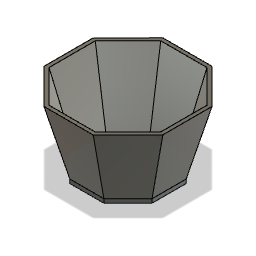
MacetaFinal (Autodesk Fusion 360 design; units mm, degrees)
Autodesk Fusion 360 part; units mm, degrees
sketch "Boceto2" plane through (0, 0, 0) normal (0, 1, 0) x (1, 0, 0)
  line L0 (0, 0) -> (35, 0)
  line L1 (35, 0) -> (59.7299, -24.7676)
  line L2 (59.7299, -24.7676) -> (59.7299, -59.7676)
  line L3 (59.7299, -59.7676) -> (34.9925, -84.5277)
  line L4 (34.9925, -84.5277) -> (-0.0075, -84.5277)
  line L5 (-0.0075, -84.5277) -> (-24.7562, -59.779)
  line L6 (-24.7562, -59.779) -> (-24.7562, -24.779)
  line L7 (0, 0) -> (-24.7562, -24.779)
  dimension "d12" = 35
  dimension "d16" = 35
  constraint coincident L0.start L7.start
  constraint horizontal L0
  constraint vertical L2
  constraint perpendicular L2 L4
  constraint vertical L6
  measures "d12" distance of L0.start L0.end
  measures "d16" distance of L3.end L4.end
extrude "Extruir1" add sketch "Boceto2" along normal blind 70 draft 15
sketch "Boceto3" plane through (0, 0, 0) normal (0, 0, 1) x (1, 0, 0)
  line L0 (33.4625, 0, 80.8319) -> (56.0342, 0, 58.2371)
  line L1 (56.0346, 0, 26.2989) -> (56.0342, 0, 58.2371)
  line L2 (56.0346, 0, 26.2989) -> (33.4695, 0, 3.6956)
  line L3 (33.4695, 0, 3.6956) -> (1.53, 0, 3.6958)
  line L4 (-21.0606, 0, 26.3095) -> (1.53, 0, 3.6958)
  line L5 (-21.0606, 0, 26.3095) -> (-21.061, 0, 58.2476)
  line L6 (-21.061, 0, 58.2476) -> (1.5231, 0, 80.8321)
  line L7 (1.5231, 0, 80.8321) -> (33.4625, 0, 80.8319)
  point P0 (34.9925, 0)
  point P1 (59.7299, 0)
  point P2 (-24.7562, 0)
  point P3 (-0.0075, 0)
  point P4 (35, 0)
  point P5 (59.7299, 0)
  point P6 (-24.7562, 0)
  dimension "d26" = 4
  dimension "d27" = 4
  dimension "d30" = 4
  dimension "d31" = 4
extrude "Extruir2" cut sketch "Boceto3" along normal blind 80 draft 15 contours L0 L1 L2 L3 L4 L5 L6 L7 in plane through (0, 0, 0) normal (0, 1, 0)
sketch "Boceto4" plane through (0, 0, 0) normal (0, -1, 0) x (1, 0, 0)
  line L0 (1.53, 3.6958) -> (-21.0606, 26.3095)
  line L1 (-21.0606, 26.3095) -> (-21.061, 58.2476)
  line L2 (-21.061, 58.2476) -> (1.5231, 80.8321)
  line L3 (1.5231, 80.8321) -> (33.4625, 80.8319)
  line L4 (33.4625, 80.8319) -> (56.0342, 58.2371)
  line L5 (56.0342, 58.2371) -> (56.0346, 26.2989)
  line L6 (56.0346, 26.2989) -> (33.4695, 3.6956)
  line L7 (33.4695, 3.6956) -> (1.53, 3.6958)
  line L8 (0, 0) -> (35, 0)
  line L9 (35, 0) -> (59.7299, 24.7676)
  line L10 (59.7299, 24.7676) -> (59.7299, 59.7676)
  line L11 (59.7299, 59.7676) -> (34.9925, 84.5277)
  line L12 (34.9925, 84.5277) -> (-0.0075, 84.5277)
  line L13 (-0.0075, 84.5277) -> (-24.7562, 59.779)
  line L14 (-24.7562, 59.779) -> (-24.7562, 24.779)
  line L15 (-24.7562, 24.779) -> (0, 0)
  line L16 (-0.0075, 84.5277) -> (34.9925, 84.5277)
  line L17 (59.7299, 59.7676) -> (59.7299, 24.7676)
  line L18 (35, 0) -> (0, 0)
  line L19 (-24.7562, 24.779) -> (-24.7562, 59.779)
  constraint coincident L12.end L13.start
  constraint coincident L11.end L12.start
  constraint coincident L10.end L11.start
  constraint coincident L9.end L10.start
  constraint coincident L8.end L9.start
  constraint coincident L8.start L15.end
  constraint coincident L14.end L15.start
  constraint coincident L13.end L14.start
extrude "Extruir3" add sketch "Boceto4" along normal blind 4 contours L0 L1 L2 L3 L4 L5 L6 L7 | L8 L9 L10 L11 L12 L13 L14 L15 L16 L17 L18 L19
sketch "Boceto5" plane through (0, -4, 0) normal (0, -1, 0) x (1, 0, 0)
  line L0 (35, 0) -> (59.7299, 24.7676)
  line L1 (59.7299, 24.7676) -> (59.7299, 59.7676)
  line L2 (59.7299, 59.7676) -> (34.9925, 84.5277)
  line L3 (34.9925, 84.5277) -> (-0.0075, 84.5277)
  line L4 (-0.0075, 84.5277) -> (-24.7562, 59.779)
  line L5 (-24.7562, 59.779) -> (-24.7562, 24.779)
  line L6 (-24.7562, 24.779) -> (0, 0)
  line L7 (0, 0) -> (35, 0)
hole "Agujero1" at (-12.3839, -4, 29.9025) direction (0, 1, 0) diameter 10 depth 35 tip angle 118
hole "Agujero2" at (47.362, -4, 54.6456) direction (0, 1, 0) diameter 10 depth 35 tip angle 118
sketch "Boceto6" plane through (0, 0, 0) normal (0, 1, 0) x (1, 0, 0)
  circle A0 centre (-12.3839, -29.9025) radius 5
  point P0 (-21.0606, -26.3095)
  point P1 (33.4625, -80.8319)
  point P2 (56.0342, -58.2371)
sketch "Boceto7" plane through (0, 0, 0) normal (0, 1, 0) x (-1, 0, 0)
  circle A0 centre (-47.362, 54.6456) radius 5
  circle A1 centre (12.3839, 29.9025) radius 5
  line L0 (-33.4625, 80.8319) -> (-56.0342, 58.2371)
  line L1 (-56.0342, 58.2371) -> (-56.0346, 26.2989)
  line L2 (-56.0346, 26.2989) -> (-33.4695, 3.6956)
  line L3 (-33.4695, 3.6956) -> (-1.53, 3.6958)
  line L4 (-1.53, 3.6958) -> (21.0606, 26.3095)
  line L5 (21.0606, 26.3095) -> (21.061, 58.2476)
  line L6 (21.061, 58.2476) -> (-1.5231, 80.8321)
  line L7 (-1.5231, 80.8321) -> (-33.4625, 80.8319)
  circle A2 centre (-31.8777, 7.539) radius 3
  circle A3 centre (-3.1148, 76.9887) radius 3
  dimension "d44" = 4.16
  dimension "d45" = 4.16
  dimension "d46" = 6
  dimension "d47" = 6
  measures "d44" distance of L2.end A2.centre
  measures "d45" distance of L6.end A3.centre
  measures "d46" diameter of A2
  measures "d47" diameter of A3
extrude "Extruir4" cut sketch "Boceto7" against normal blind 4 contours A2
sketch "Boceto8" plane through (0, 0, 0) normal (0, 1, 0) x (1, 0, 0)
  circle A0 centre (3.1119, -76.9867) radius 3
  dimension "d51" = 6
  measures "d51" diameter of A0
extrude "Extruir5" cut sketch "Boceto8" against normal blind 4
sketch "Boceto9" plane through (0, 0, 0) normal (0, 1, 0) x (-1, 0, 0)
  circle A0 centre (-3.1119, 76.9867) radius 3
  circle A1 centre (-31.8777, 7.539) radius 3
  circle A2 centre (-47.362, 54.6456) radius 5
  circle A3 centre (12.3839, 29.9025) radius 5
  line L0 (-33.4625, 80.8319) -> (-56.0342, 58.2371)
  line L1 (-56.0342, 58.2371) -> (-56.0346, 26.2989)
  line L2 (-56.0346, 26.2989) -> (-33.4695, 3.6956)
  line L3 (-33.4695, 3.6956) -> (-1.53, 3.6958)
  line L4 (-1.53, 3.6958) -> (21.0606, 26.3095)
  line L5 (21.0606, 26.3095) -> (21.061, 58.2476)
  line L6 (21.061, 58.2476) -> (-1.5231, 80.8321)
  line L7 (-1.5231, 80.8321) -> (-33.4625, 80.8319)
  circle A4 centre (-47.362, 54.6456) radius 5
  constraint concentric A2 A4
extrude "Extruir6" add sketch "Boceto9" against normal blind 4 contours A2 A4
extrude "Extruir7" add sketch "Boceto6" against normal blind 4
sketch "Boceto10" plane through (0, 0, 0) normal (0, 1, 0) x (-1, 0, 0)
  circle A0 centre (-3.1119, 76.9867) radius 3
  circle A1 centre (-31.8777, 7.539) radius 3
  line L0 (-33.4625, 80.8319) -> (-56.0342, 58.2371)
  line L1 (-56.0342, 58.2371) -> (-56.0346, 26.2989)
  line L2 (-56.0346, 26.2989) -> (-33.4695, 3.6956)
  line L3 (-33.4695, 3.6956) -> (-1.53, 3.6958)
  line L4 (-1.53, 3.6958) -> (21.0606, 26.3095)
  line L5 (21.0606, 26.3095) -> (21.061, 58.2476)
  line L6 (21.061, 58.2476) -> (-1.5231, 80.8321)
  line L7 (-1.5231, 80.8321) -> (-33.4625, 80.8319)
  line L8 (-56.0342, 58.2371) -> (-51.114, 56.1995)
  circle A2 centre (-51.114, 56.1995) radius 5
  dimension "d58" = 5.3255
  dimension "d59" = 10
  constraint coincident L0.end L1.start
  constraint coincident L8.end A2.centre
  measures "d58" distance of L0.end L8.end
  measures "d59" diameter of A2
extrude "Extruir8" cut sketch "Boceto10" against normal blind 10 contours L0 L1 A2
sketch "Boceto11" plane through (0, 0, 0) normal (0, 1, 0) x (1, 0, 0)
  circle A0 centre (-16.1401, -28.3484) radius 5
  dimension "d63" = 10
  measures "d63" diameter of A0
extrude "Extruir9" cut sketch "Boceto11" against normal blind 10
